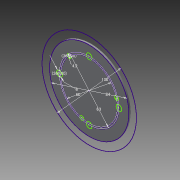
# Autodesk Inventor part: plate2
Saved by Autodesk Inventor 2015 (Build 190159000, 159)
## iProperties
Created: 2016-05-10
Part Number: plate2
Material: 一般
Document SubType Name: Modeling
Designer: Ryo
Density: 1 g/cm^3
Appearance: 既定
Author: Ryo
Autodesk Inventor part; units mm, degrees
ref_plane "YZ Plane" through (0, 0, 0) normal (1, 0, 0) x (0, 1, 0)
ref_plane "XZ Plane" through (0, 0, 0) normal (0, 1, 0) x (-1, 0, 0)
ref_plane "XY Plane" through (0, 0, 0) normal (0, 0, 1) x (1, 0, 0)
sketch "スケッチ1" plane through (0, 0, 0) normal (0, 1, 0) x (-1, 0, 0)
  circle A0 centre (0, 0) radius 50
  circle A1 centre (0, 0) radius 31.5
  circle A2 centre (31.5, 0) radius 3
  circle A3 centre (0, 31.5) radius 3
  circle A4 centre (-31.5, 0) radius 3
  circle A5 centre (0, -31.5) radius 3
  circle A6 centre (0, 0) radius 30
  circle A7 centre (21.2132, 21.2132) radius 2.1
  circle A8 centre (-28.9778, 7.7646) radius 2.1
  circle A9 centre (7.7646, -28.9778) radius 2.1
  circle A10 centre (0, 0) radius 42
  dimension "d1" = 63
  dimension "d0" = 100
  dimension "d2" = 6
  dimension "d5" = 360
  dimension "d7" = 60
  dimension "d8" = 4.2
  dimension "d11" = 360
  dimension "d17" = 84
  constraints: 10 centre point, 4 coincident, 1 horizontal alignment, 18 other
  measures "d0" diameter of A0
  measures "d2" diameter of A2
  measures "d7" diameter of A6
  measures "d8" diameter of A7
  measures "d17" diameter of A10
extrude "押し出し1" add sketch "スケッチ1" along normal blind 2 contours A0 | A2 A6 A7 A1 | A1 A9 A6 A2 | A2 A6 A9 A5 A4 A8 A3 A7 | A7 A6 A3 A1 | A1 A5 A6 A9 | A3 A6 A8 A1 | A1 A4 A6 A5 | A8 A6 A4 A1 | A10
extrude "押し出し2" cut sketch "スケッチ1" along normal blind 2 contours A1 A2 A6 | A1 A2 | A7 A6 A1 | A1 A7 | A6 A2 | A9 A1 | A1 A9 A6 | A7 A6 | A6 A9 | A3 A6 A1 | A1 A3 | A5 A1 | A1 A5 A6 | A3 A6 | A6 A5 | A8 A6 A1 | A1 A8 | A4 A1 | A1 A4 A6 | A8 A6 | A6 A4
extrude "押し出し3" cut sketch "スケッチ1" along normal blind 10 contours A0
extrude "押し出し4" add sketch "スケッチ1" along normal blind 2 contours A1 A2 A6 | A1 A2 | A6 A2 | A3 A6 A1 | A1 A3 | A5 A1 | A1 A5 A6 | A3 A6 | A6 A5 | A4 A1 | A1 A4 A6 | A6 A4
